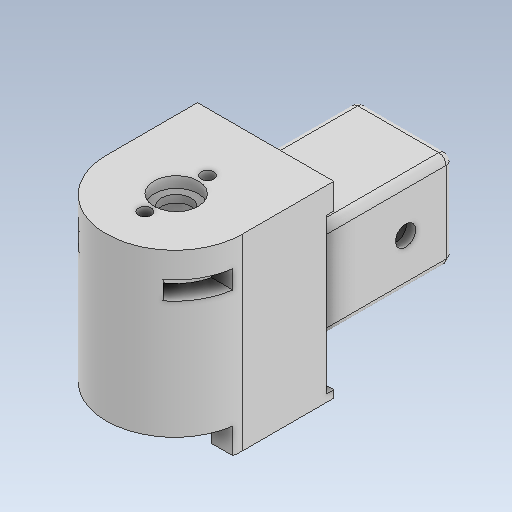
# Autodesk Inventor part: 5_Connettore_sup_inf
Saved by Autodesk Inventor 2020.2 (Build 242310000, 310)
## iProperties
Created: 2019-10-13
Part Number: 5_Connettore_sup_inf
Material: PLA(Stampato)
Document SubType Name: Modeling
Designer: socci
Density: 0.988 g/cm^3
Appearance: Default(1)
Mass: 64.0108 g
Surface Area: 242.78 cm^2
Volume: 64.7882 cm^3
Author: socci
Autodesk Inventor part; units mm, degrees
note: some values were not read from the file. Chosen so that the rebuilt part matches the saved one: direction of "Foro4"; direction of "Foro5"; direction of "Foro6"; direction of "Foro7".
ref_plane "YZ Plane" through (0, 0, 0) normal (1, 0, 0) x (0, 1, 0)
ref_plane "XZ Plane" through (0, 0, 0) normal (0, 1, 0) x (-1, 0, 0)
ref_plane "XY Plane" through (0, 0, 0) normal (0, 0, 1) x (1, 0, 0)
sketch "Schizzo1" plane through (0, 0, 0) normal (0, 0, 1) x (1, 0, 0)
  line L0 (9, 6) -> (9, -6)
  line L1 (6, -9) -> (-6, -9)
  line L2 (-9, -6) -> (-9, 6)
  line L3 (-6, 9) -> (6, 9)
  arc A0 (-6, 9) -> (-9, 6) centre (-6, 6) ccw
  arc A1 (-9, -6) -> (-6, -9) centre (-6, -6) ccw
  arc A2 (6, -9) -> (9, -6) centre (6, -6) ccw
  arc A3 (9, 6) -> (6, 9) centre (6, 6) ccw
  point P0 (0, 0)
  point P1 (0, 0)
  point P2 (9, 9)
  point P3 (9, -9)
  point P4 (-9, -9)
  point P5 (-9, 9)
  dimension "d0" = 18
  dimension "d72" = 3
  constraints: 8 end point, 8 point on circle, 8 point on line, 8 tangent, 4 centre point, 3 equal radius, 1 coincident, 9 other
  measures "d0" distance of point (9, 9) point (9, -9)
  measures "d72" radius of A0
extrude "Estrusione1" add sketch "Schizzo1" against normal blind 40
sketch "Schizzo2" plane through (0, 0, 0) normal (0, 0, 1) x (1, 0, 0)
  line L0 (18.5, -23) -> (-18.5, -23)
  line L1 (-18.5, -23) -> (-18.5, 23)
  line L2 (-18.5, 23) -> (18.5, 23)
  line L3 (18.5, 23) -> (18.5, -23)
  line L4 (18.5, -23) -> (-18.5, 23) construction
  line L5 (-18.5, -23) -> (18.5, 23) construction
  point P0 (0, 0)
  dimension "d3" = 46
  dimension "d4" = 37
  constraints: 12 end point, 3 midpoint, 2 parallel, 1 horizontal, 1 perpendicular
  measures "d3" distance of L0.end L1.end
  measures "d4" distance of L1.end L2.end
extrude "Estrusione2" add sketch "Schizzo2" along normal blind 21
sketch "Schizzo3" plane through (-18.5, 23, 0) normal (0, 1, 0) x (1, 0, 0)
  line L0 (18.5, 0) -> (18.5, -22.5)
  line L1 (18.5, 0) -> (41, 0) construction
  circle A0 centre (18.5, -22.5) radius 12.8
  dimension "d7" = 22.5
  dimension "d8" = 90
  dimension "d9" = 25.6
  constraints: 4 end point, 1 centre point, 1 coincident, 1 horizontal, 1 perpendicular, 1 vertical
  measures "d7" distance of L0.start L0.end
  measures "d8" angle of L0 L1
  measures "d9" diameter of A0
extrude "Estrusione3" cut sketch "Schizzo3" against normal blind 46
sketch "Schizzo7" plane through (-18.5, 23, 0) normal (0, 1, 0) x (1, 0, 0)
  arc A0 (31.2118, -21) -> (5.7882, -21) centre (18.5, -22.5) ccw projected
  line L0 (0, 0) -> (0, -22.5)
  circle A1 centre (18.5, -22.5) radius 18.5
  line L1 (18.5, 0) -> (4.5, 0)
  line L2 (37, 0) -> (0, 0) projected
  line L3 (18.5, 0) -> (32.5, 0) construction
  line L4 (4.5, 0) -> (4.5, -10.4066)
  point P0 (16.5, -34.839)
  point P1 (20.5, -34.839)
  dimension "d73" = 37
  dimension "d74" = 14
  dimension "d75" = 180
  dimension "d76" = 90
  constraints: 8 end point, 2 collinear, 1 coincident, 1 horizontal, 3 other
  measures "d74" distance of L1.start L1.end
  measures "d75" angle of L1 L3
  measures "d76" angle of L4 L1
extrude "Estrusione7" [suppressed]
sketch "Schizzo8" plane through (0, 23, 22.5) normal (0, 1, 0) x (1, 0, 0)
  line L0 (-6, 22.5) -> (6, 22.5) projected
  arc A0 (12.7118, 1.5) -> (-12.7118, 1.5) centre (0, 0) ccw projected
  circle A1 centre (0, 0) radius 18.5
  line L1 (0, 22.5) -> (14, 22.5)
  line L2 (0, 22.5) -> (14, 22.5) construction
  line L3 (14, 22.5) -> (14, 12.0934)
  line L4 (-18.5, 22.5) -> (18.5, 22.5) projected
  line L5 (14, 22.5) -> (18.5, 22.5)
  line L6 (18.5, 22.5) -> (18.5, 0)
  point P0 (-9, 22.5)
  point P1 (9, 22.5)
  point P2 (2, -12.339)
  point P3 (-2, -12.339)
  point P4 (-14, 22.5)
  dimension "d35" = 37
  dimension "d36" = 14
  dimension "d38" = 90
  constraints: 10 end point, 2 collinear, 2 horizontal, 2 point on circle, 1 centre point, 1 coincident, 1 perpendicular
  measures "d35" diameter of A1
  measures "d36" distance of L1.start L1.end
  measures "d38" angle of L1 L3
extrude "Estrusione8" [suppressed]
sketch "Schizzo14" plane through (0, 0, 0) normal (0, 0, -1) x (-1, 0, 0)
  line L0 (-11, 13) -> (11, 13)
  line L1 (13, 11) -> (13, -11)
  line L2 (11, -13) -> (-11, -13)
  line L3 (-13, -11) -> (-13, 11)
  arc A0 (11, -13) -> (13, -11) centre (11, -11) ccw
  arc A1 (-13, -11) -> (-11, -13) centre (-11, -11) ccw
  arc A2 (13, 11) -> (11, 13) centre (11, 11) ccw
  arc A3 (-11, 13) -> (-13, 11) centre (-11, 11) ccw
  line L4 (-9.382, 10.5) -> (9.382, 10.5)
  line L5 (10.5, 9.382) -> (10.5, -9.382)
  line L6 (9.382, -10.5) -> (-9.382, -10.5)
  line L7 (-10.5, -9.382) -> (-10.5, 9.382)
  arc A4 (-10.1273, 10.8333) -> (-10.8333, 10.1273) centre (-10.5, 10.5) ccw
  arc A5 (-10.1273, 10.8333) -> (-9.382, 10.5) centre (-9.382, 11.5) ccw
  arc A6 (-10.5, 9.382) -> (-10.8333, 10.1273) centre (-11.5, 9.382) ccw
  arc A7 (10.8333, 10.1273) -> (10.1273, 10.8333) centre (10.5, 10.5) ccw
  arc A8 (9.382, 10.5) -> (10.1273, 10.8333) centre (9.382, 11.5) ccw
  arc A9 (10.8333, 10.1273) -> (10.5, 9.382) centre (11.5, 9.382) ccw
  arc A10 (10.1273, -10.8333) -> (10.8333, -10.1273) centre (10.5, -10.5) ccw
  arc A11 (10.1273, -10.8333) -> (9.382, -10.5) centre (9.382, -11.5) ccw
  arc A12 (10.5, -9.382) -> (10.8333, -10.1273) centre (11.5, -9.382) ccw
  arc A13 (-10.8333, -10.1273) -> (-10.1273, -10.8333) centre (-10.5, -10.5) ccw
  arc A14 (-9.382, -10.5) -> (-10.1273, -10.8333) centre (-9.382, -11.5) ccw
  arc A15 (-10.8333, -10.1273) -> (-10.5, -9.382) centre (-11.5, -9.382) ccw
  point P0 (0, 0)
  point P1 (0, 0)
  point P2 (-10.5, 10.5)
  point P3 (10.5, 10.5)
  point P4 (10.5, -10.5)
  point P5 (-10.5, -10.5)
  point P6 (0, 0)
  point P7 (-13, 13)
  point P8 (13, 13)
  point P9 (13, -13)
  point P10 (-13, -13)
  point P11 (0, 0)
  point P12 (-10, 10.5)
  point P13 (-10.5, 10)
  point P14 (10.5, 10)
  point P15 (10, 10.5)
  point P16 (10, -10.5)
  point P17 (10.5, -10)
  point P18 (-10.5, -10)
  point P19 (-10, -10.5)
  dimension "d77" = 21
  dimension "d78" = 26
  dimension "d102" = 2
  dimension "d110" = 1
  dimension "d112" = 1
  dimension "d114" = 1
  dimension "d116" = 1
  constraints: 40 point on circle, 24 tangent, 16 centre point, 16 end point, 16 point on line, 5 equal radius, 3 coincident, 19 other
  measures "d77" distance of point (-10.5, -10.5) point (-10.5, 10.5)
  measures "d78" distance of point (-13, -13) point (-13, 13)
  measures "d102" radius of A2
  measures "d110" radius of A5
  measures "d112" radius of A8
  measures "d114" radius of A11
  measures "d116" radius of A14
extrude "Estrusione10" add sketch "Schizzo14" along normal blind 40
sketch "Schizzo15" plane through (-13, 13, 0) normal (0, 1, 0) x (1, 0, 0)
  line L0 (13, 0) -> (13, 13)
  line L1 (13, 0) -> (26, 0) construction
  dimension "d82" = 13
  dimension "d83" = 90
  constraints: 4 end point, 1 horizontal, 1 perpendicular, 1 vertical
  measures "d82" distance of L0.start L0.end
  measures "d83" angle of L1 L0
hole "Foro4" at (0, 13, -13) direction (0, -1, 0) diameter 5.5 depth 26 clearance for "Vite a testa esagonale" size "M5" standard "ANSI - Profilo M Metrico"
sketch "Schizzo16" plane through (13, -11, 0) normal (1, 0, 0) x (0, 0, -1)
  line L0 (0, 11) -> (27, 11)
  line L1 (0, 11) -> (27, 11) construction
  dimension "d91" = 27
  dimension "d92" = 0
  constraints: 4 end point, 2 horizontal, 1 collinear
  measures "d91" distance of L0.start L0.end
  measures "d92" distance between parallel lines of L0 L1
hole "Foro5" at (13, 0, -27) direction (-1, 0, 0) diameter 5.5 depth 26 clearance for "Vite a testa esagonale" size "M5" standard "ANSI - Profilo M Metrico"
fillet "Raccordo1" radius 2 1 edges at (0, -13, -40)
fillet "Raccordo2" radius 2 1 edges at (-9, 0, -40)
fillet "Raccordo3" radius 3 1 edges at (-13, 0, 0)
sketch "Schizzo17" plane through (0, 0, 0) normal (0, 0, -1) x (-1, 0, 0)
  point P0 (0, 0)
sketch "Schizzo18" plane through (0, 0, 0) normal (0, 0, -1) x (-1, 0, 0)
  line L0 (18.5, -23) -> (12.7118, -23) projected
  line L1 (18.5, 23) -> (18.5, -23) projected
  line L2 (-18.5, -23) -> (-18.5, 23) projected
  line L3 (18.5, -23) -> (-18.5, -23)
  line L4 (-18.5, -23) -> (-18.5, -21)
  line L5 (-18.5, -21) -> (18.5, -21)
  line L6 (18.5, -21) -> (18.5, -23)
  line L7 (12.7118, -23) -> (-12.7118, -23) projected
  line L8 (12.7118, 23) -> (18.5, 23) projected
  line L9 (18.5, 23) -> (-18.5, 23)
  line L10 (-18.5, 23) -> (-18.5, 21)
  line L11 (-18.5, 21) -> (18.5, 21)
  line L12 (18.5, 21) -> (18.5, 23)
  point P0 (0, 0)
  dimension "d104" = 2
  dimension "d105" = 2
  constraints: 16 end point, 4 parallel, 2 collinear, 2 perpendicular
  measures "d104" distance of L2.start L4.end
  measures "d105" distance of L10.end L2.end
extrude "Estrusione11" add sketch "Schizzo18" along normal blind 2 contours L0 L3 L2 L5 L1 | L11 L2 L9 L8 L1
sketch "Schizzo19" plane through (0, 23, 22.5) normal (0, 1, 0) x (1, 0, 0)
  line L0 (-18.5, 24.5) -> (18.5, 24.5) projected
  line L1 (0, 24.5) -> (0, 12.8)
  arc A0 (12.7118, 1.5) -> (-12.7118, 1.5) centre (0, 0) ccw projected
  line L2 (0, 12.8) -> (0, -13.75)
  line L3 (0, -13.75) -> (0, -18.75)
  line L4 (0, -13.75) -> (5, -13.75) construction
  line L5 (18.5, 24.5) -> (-18.5, 24.5)
  line L6 (-18.5, 24.5) -> (-18.5, -18.75)
  line L7 (-18.5, -18.75) -> (18.5, -18.75)
  line L8 (18.5, -18.75) -> (18.5, 24.5)
  point P0 (0, 22.5)
  dimension "d117" = 5
  dimension "d118" = 90
  constraints: 16 end point, 3 equal length, 3 vertical, 2 midpoint, 2 perpendicular, 1 horizontal, 1 point on circle
  measures "d117" distance of L2.end L3.end
  measures "d118" angle of L3 L4
extrude "Estrusione12" add sketch "Schizzo19" along normal blind 5
sketch "Schizzo20" plane through (0, 28, 22.5) normal (0, 1, 0) x (1, 0, 0)
  arc A0 (12.7118, 1.5) -> (-12.7118, 1.5) centre (0, 0) ccw construction
  circle A1 centre (0, 0) radius 12.8 construction
  arc A2 (12.7118, 1.5) -> (-12.7118, 1.5) centre (0, 0) ccw projected
  line L0 (0, 12.8) -> (0, 0.2)
  line L1 (0, 12.8) -> (12.6, 12.8) construction
  line L2 (0, -8.3) -> (0, 8.7)
  line L3 (0, -8.3) -> (17, -8.3) construction
  point P0 (0, 22.5)
  dimension "d151" = 12.6
  dimension "d152" = 90
  dimension "d153" = 17
  dimension "d154" = 90
  constraints: 8 end point, 4 coincident, 2 horizontal, 2 perpendicular, 2 point on circle, 2 vertical, 1 centre point, 1 midpoint
  measures "d151" distance of L0.end L0.start
  measures "d152" angle of L0 L1
  measures "d153" distance of L2.start L2.end
  measures "d154" angle of L3 L2
hole "Foro6" at (0, 28, 30.8) at (0, 28, 13.8) direction (0, -1, 0) diameter 3.5 depth 5 clearance for "Vite a testa piana" size "M3" standard "ANSI - Profilo M Metrico"
sketch "Schizzo21" plane through (0, 28, 22.5) normal (0, 1, 0) x (1, 0, 0)
  circle A0 centre (0, -8.3) radius 1.75 projected
  circle A1 centre (0, 8.7) radius 1.75 projected
  line L0 (0, -8.3) -> (0, 8.7)
  circle A2 centre (0, 0.2) radius 3.5 construction
  point P0 (0, 22.5)
  point P1 (0, 0.2)
  point P2 (0, 0.2)
  dimension "d155" = 7
  constraints: 2 coincident, 2 end point, 1 centre point, 1 midpoint, 1 vertical
  measures "d155" diameter of A2
hole "Foro7" at (0, 28, 22.3) direction (0, -1, 0) diameter 8 depth 5
sketch "Schizzo22" plane through (0, 28, 22.5) normal (0, 1, 0) x (1, 0, 0)
  circle A0 centre (0, 0.2) radius 4 projected
  circle A1 centre (0, 0.2) radius 5 construction
  point P0 (0, 22.5)
  dimension "d156" = 10
  constraints: 2 coincident, 1 centre point
  measures "d156" diameter of A1
hole "Foro8" at (0, 28, 22.3) direction (0, -1, 0) diameter 12 depth 3
sketch "Schizzo23" plane through (0, 23, 22.5) normal (0, -1, 0) x (1, 0, 0)
  line L0 (-18.5, 18.75) -> (18.5, 18.75)
  line L1 (18.5, -1.5) -> (-18.5, -1.5)
  line L2 (-18.5, -1.5) -> (-18.5, 18.75)
  line L3 (-18.5, -1.5) -> (-12.7118, -1.5) projected
  line L4 (12.7118, -1.5) -> (18.5, -1.5) projected
  line L5 (12.7118, -1.5) -> (18.5, -1.5)
  line L6 (-12.7118, -1.5) -> (-18.5, -1.5)
  line L7 (-18.5, 18.75) -> (18.5, 18.75) projected
  line L8 (-18.5, 18.75) -> (18.5, 18.75)
  line L9 (18.5, 18.75) -> (18.5, -1.5)
  arc A0 (-12.7118, -1.5) -> (12.7118, -1.5) centre (0, 0) ccw projected
  circle A1 centre (0, 0) radius 12.8
  point P0 (0, -22.5)
  constraints: 14 end point, 3 collinear, 1 centre point, 1 coincident, 1 parallel, 1 perpendicular
extrude "Estrusione13" add sketch "Schizzo23" along normal up to surface (46 mm away) contours L0 L9 L1 A1 L2
sketch "Schizzo24" plane through (-18.5, 28, 41.25) normal (0, 0, 1) x (1, 0, 0)
  line L0 (37, -7) -> (0, -7) projected
  line L1 (0, -49) -> (37, -49) projected
  line L2 (7.5, -12) -> (29.5, -12) projected
  line L3 (29.5, -44) -> (7.5, -44) projected
  line L4 (0, -7) -> (37, -7) projected
  line L5 (37, -7) -> (0, -7)
  line L6 (0, -7) -> (0, -12)
  line L7 (0, -12) -> (37, -12)
  line L8 (37, -12) -> (37, -7)
  line L9 (0, -51) -> (0, 0) projected
  line L10 (37, -49) -> (0, -49)
  line L11 (0, -49) -> (0, -44)
  line L12 (0, -44) -> (37, -44)
  line L13 (37, -44) -> (37, -49)
  line L14 (37, -49) -> (0, -49) projected
  line L15 (37, -49) -> (0, -49)
  line L16 (0, -49) -> (0, -51)
  line L17 (0, -51) -> (37, -51)
  line L18 (37, -51) -> (37, -49)
  point P0 (18.5, -28)
  point P1 (29.5, -44)
  point P2 (7.5, -44)
  point P3 (0, -44)
  point P4 (7.5, -12)
  point P5 (29.5, -12)
  point P6 (0, -51)
  constraints: 24 end point, 7 equal length, 5 perpendicular
extrude "Estrusione14" cut sketch "Schizzo24" against normal blind 16
sketch "Schizzo25" plane through (-18.5, 21, 41.25) normal (0, -1, 0) x (1, 0, 0)
  arc A0 (5.7882, -20.25) -> (5.7882, -20.25) centre (18.5, -18.75) ccw projected
  line L0 (18.5, -5.95) -> (18.5, -3.95)
  line L1 (0, 0) -> (37, 0) projected
  line L2 (18.5, -5.95) -> (20.5, -5.95) construction
  line L3 (37, 0) -> (37, -43.25) projected
  line L4 (0, 0) -> (37, 0)
  line L5 (37, 0) -> (37, -3.95)
  line L6 (37, -3.95) -> (0, -3.95)
  line L7 (0, -3.95) -> (0, 0)
  point P0 (18.5, -41.25)
  dimension "d146" = 2
  dimension "d147" = 90
  constraints: 12 end point, 4 perpendicular, 2 parallel, 1 horizontal, 1 midpoint, 1 point on circle
  measures "d146" distance of L0.end L0.start
  measures "d147" angle of L2 L0
extrude "Estrusione15" add sketch "Schizzo25" along normal up to surface (5 mm away) contours L1 L3 L6 L7
full round fillet "Raccordo4" first side at (18.5, -5.3333, 8.4167) centre faces at (6.1667, -1.3333, 41.25) second side at (-18.5, -5.3333, 8.4167)
